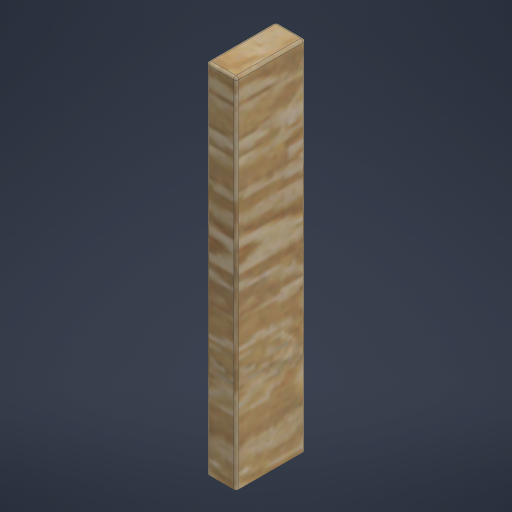
# Autodesk Inventor part: Barren Stand
Saved by Autodesk Inventor 2024.1 (Build 281209000, 209)
## iProperties
Created: 2024-11-18
Part Number: Barren Stand
Material: Generic
Document SubType Name: Modeling
Designer: Designer
Density: 1 g/cm^3
Appearance: Default
Author: Designer
Autodesk Inventor part; units mm, degrees
ref_plane "YZ Plane" through (0, 0, 0) normal (1, 0, 0) x (0, 1, 0)
ref_plane "XZ Plane" through (0, 0, 0) normal (0, 1, 0) x (-1, 0, 0)
ref_plane "XY Plane" through (0, 0, 0) normal (0, 0, 1) x (1, 0, 0)
sketch "Sketch1" plane through (0, 0, 0) normal (0, 1, 0) x (-1, 0, 0)
  line L0 (0, 0) -> (38.1, 0)
  line L1 (38.1, 0) -> (38.1, 88.9)
  line L2 (38.1, 88.9) -> (0, 88.9)
  line L3 (0, 88.9) -> (0, 0)
  dimension "d0" = 38.1
  dimension "d1" = 88.9
  constraints: 8 end point, 2 parallel, 1 horizontal, 1 perpendicular
  measures "d0" distance of L0.start L0.end
  measures "d1" distance of L2.end L0.start
extrude "Extrusion1" add sketch "Sketch1" along normal blind 457.2
fillet "Fillet1" radius 3.175 8 edges at (0, 228.6, 88.9) (-38.1, 228.6, 88.9) (0, 228.6, 0) (-38.1, 228.6, 0) (-19.05, 457.2, 0) (0, 457.2, 44.45) (-38.1, 457.2, 44.45) (-19.05, 457.2, 88.9)
body "Solid1"
